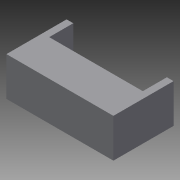
# Autodesk Inventor part: IR Cover
Saved by Autodesk Inventor 2014 SP2 (Build 180246200, 246)
## iProperties
Created: 2015-08-22
Part Number: IR Cover
Material: Generic
Document SubType Name: Modeling
Designer: Devon
Density: 1 g/cm^3
Appearance: Default
Author: Devon
Autodesk Inventor part; units mm, degrees
ref_plane "YZ Plane" through (0, 0, 0) normal (1, 0, 0) x (0, 1, 0)
ref_plane "XZ Plane" through (0, 0, 0) normal (0, 1, 0) x (-1, 0, 0)
ref_plane "XY Plane" through (0, 0, 0) normal (0, 0, 1) x (1, 0, 0)
sketch "Sketch1" plane through (0, 0, 0) normal (0, 1, 0) x (-1, 0, 0)
  line L0 (0, 0) -> (50.8, 0)
  line L1 (50.8, 0) -> (50.8, 28.575)
  line L2 (50.8, 28.575) -> (0, 28.575)
  line L3 (0, 28.575) -> (0, 0)
  line L4 (0, 28.575) -> (50.8, 28.575)
  line L5 (50.8, 28.575) -> (50.8, 25.4)
  line L6 (47.625, 25.4) -> (3.175, 25.4)
  line L7 (0, 25.4) -> (0, 28.575)
  line L8 (47.625, 25.4) -> (47.625, 0)
  line L9 (47.625, 0) -> (50.8, 0)
  line L10 (50.8, 0) -> (50.8, 25.4)
  line L11 (0, 0) -> (3.175, 0)
  line L12 (3.175, 0) -> (3.175, 25.4)
  line L13 (0, 25.4) -> (0, 0)
  line L14 (25.4, 0) -> (27.94, 0)
  line L15 (25.4, 0) -> (22.86, 0)
  line L16 (22.86, 0) -> (27.94, 0)
  line L17 (27.94, 0) -> (27.94, 17.78)
  line L18 (22.86, 17.78) -> (22.86, 0)
  arc A0 (27.94, 17.78) -> (22.86, 17.78) centre (25.4, 17.78) ccw
  line L19 (3.175, 0) -> (6.985, 0)
  circle A1 centre (6.985, 6.477) radius 1.524
  line L20 (47.625, 0) -> (43.815, 0)
  circle A2 centre (43.815, 6.477) radius 1.524
  dimension "d0" = 50.8
  dimension "d1" = 28.575
  dimension "d2" = 3.175
  dimension "d3" = 3.175
  dimension "d4" = 3.175
  dimension "d5" = 2.54
  dimension "d6" = 2.54
  dimension "d11" = 3.048
  dimension "d12" = 3.81
  constraints: 42 end point, 7 parallel, 6 point on line, 4 horizontal, 4 perpendicular, 3 centre point, 2 point on circle, 1 midpoint
  measures "d0" distance of L2.end L1.end
  measures "d1" distance of L1.end L0.end
  measures "d2" distance of L4.end L5.end
  measures "d3" distance of L9.end L8.end
  measures "d4" distance of L6.end L13.start
  measures "d5" distance of L14.start L14.end
  measures "d6" distance of L14.start L15.end
  measures "d11" diameter of A1
  measures "d12" distance of L8.end L20.end
extrude "Extrusion1" add sketch "Sketch1" along normal blind 3.175 contours L3 L2 L1 L0 L8 L6 L12 | L12 L6 L8 L0 L17 A0 L18
sketch "Sketch2" plane through (0, 3.175, 0) normal (0, 1, 0) x (1, 0, 0)
  line L0 (-27.94, 0) -> (-50.8, 0) projected
  line L1 (-50.8, 0) -> (-50.8, -28.575) projected
  line L2 (0, -28.575) -> (0, 0) projected
  line L3 (0, -28.575) -> (-50.8, -28.575)
  line L4 (-50.8, -28.575) -> (-50.8, -25.4)
  line L5 (-47.625, -25.4) -> (-3.175, -25.4)
  line L6 (0, -25.4) -> (0, -28.575)
  line L7 (-47.625, -25.4) -> (-47.625, 0)
  line L8 (-47.625, 0) -> (-50.8, 0)
  line L9 (-50.8, 0) -> (-50.8, -25.4)
  line L10 (0, 0) -> (-3.175, 0)
  line L11 (-3.175, 0) -> (-3.175, -25.4)
  line L12 (0, -25.4) -> (0, 0)
  dimension "d15" = 3.175
  dimension "d16" = 3.175
  dimension "d17" = 3.175
  constraints: 20 end point, 4 parallel, 2 horizontal, 2 perpendicular, 2 point on line
  measures "d15" distance of L3.end L4.end
  measures "d16" distance of L8.end L7.end
  measures "d17" distance of L5.end L12.start
extrude "Extrusion2" add sketch "Sketch2" along normal blind 15.24
sketch "Sketch3" plane through (-3.175, 3.175, 25.4) normal (0, 0, -1) x (-1, 0, 0)
  line L0 (44.45, 0) -> (44.45, 15.24) projected
  line L1 (0, 15.24) -> (44.45, 15.24)
  line L2 (44.45, 15.24) -> (44.45, 12.065)
  line L3 (44.45, 12.065) -> (0, 12.065)
  line L4 (0, 12.065) -> (0, 15.24)
  point P0 (-3.175, -3.175)
  dimension "d20" = 3.175
  constraints: 8 end point, 2 parallel, 1 horizontal, 1 perpendicular, 1 point on line
  measures "d20" distance of L1.end L2.end
extrude "Extrusion3" add sketch "Sketch3" along normal blind 13.97
body "Solid1"
